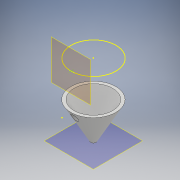
# Autodesk Inventor part: EMBOUT
Saved by Autodesk Inventor 2018 (Build 220112000, 112)
## iProperties
Created: 2018-05-14
Part Number: EMBOUT
Material: Générique
Document SubType Name: Modeling
Designer: Dimitri
Density: 1 g/cm^3
Appearance: Par défaut
Author: Dimitri
Autodesk Inventor part; units mm, degrees
ref_plane "YZ Plane" through (0, 0, 0) normal (1, 0, 0) x (0, 1, 0)
ref_plane "XZ Plane" through (0, 0, 0) normal (0, 1, 0) x (-1, 0, 0)
ref_plane "XY Plane" through (0, 0, 0) normal (0, 0, 1) x (1, 0, 0)
sketch "Esquisse1" plane through (0, 0, 0) normal (0, 0, 1) x (1, 0, 0)
  circle A0 centre (0, 0) radius 12.5
  dimension "d0" = 25
  constraints: 1 centre point, 1 coincident
  measures "d0" diameter of A0
extrude "Extrusion1" add sketch "Esquisse1" along normal blind 20
shell "Coque1" thickness 1.5 removed faces 1 at (2.488, -2.432, 20)
ref_plane "Plan de construction1" through (0, 0, -20) normal (0, 0, -1) x (-1, 0, 0)
sketch "Esquisse2" plane through (0, 0, -20) normal (0, 0, -1) x (-1, 0, 0)
  circle A0 centre (0, 0) radius 1.5
  dimension "d5" = 3
  constraints: 1 centre point, 1 coincident
  measures "d5" diameter of A0
loft "Lissage1" add profiles "Esquisse2" section 2 edges at (-12.5, 0, 0)
shell "Coque2" thickness 1.5 removed faces 1 at (0.3952, -0.1996, -20)
sketch "Esquisse3" plane through (0, 0, -20) normal (0, 0, -1) x (-1, 0, 0)
  circle A0 centre (0, 0) radius 1.1
  dimension "d11" = 2.2
  constraints: 1 centre point, 1 coincident
  measures "d11" diameter of A0
extrude "Extrusion2" cut sketch "Esquisse3" against normal blind 10
sketch "Esquisse4" plane through (0, 0, 20) normal (0, 0, 1) x (1, 0, 0)
  circle A0 centre (0, 0) radius 12.5 projected
  point P0 (0, -12.5)
  constraints: 1 vertical alignment, 1 other
ref_plane "Plan de construction2" through (0, -12.5, 20) normal (0, -1, 0) x (1, 0, 0)
sketch "Esquisse5" plane through (0, -12.5, 20) normal (0, -1, 0) x (1, 0, 0)
  circle A0 centre (0, -23.4729) radius 1
  circle A1 centre (0, -23.4729) radius 1.5
  point P0 (0, -20)
  dimension "d14" = 2
  dimension "d15" = 3
  constraints: 2 centre point, 1 coincident
  measures "d14" diameter of A0
  measures "d15" diameter of A1
extrude "Extrusion3" add sketch "Esquisse5" along normal mid plane 10
sketch "Esquisse6" plane through (0, -17.5, -3.4729) normal (0, -1, 0) x (1, 0, 0)
  circle A0 centre (0, 0) radius 1
  point P0 (0, 3.4729)
  constraints: 1 centre point
extrude "Extrusion4" cut sketch "Esquisse6" against normal blind 15
sketch "Esquisse7" plane through (0, -17.5, -3.4729) normal (0, -1, 0) x (1, 0, 0)
  point P0 (0, 3.4729)
sketch "Esquisse8" plane through (0, -17.5, -3.4729) normal (0, -1, 0) x (1, 0, 0)
  circle A0 centre (0, 0) radius 1 projected
  circle A1 centre (0, 0) radius 2
  point P0 (0, 3.4729)
  dimension "d20" = 4
  constraints: 1 centre point, 1 coincident
  measures "d20" diameter of A1
extrude "Extrusion5" cut sketch "Esquisse8" against normal blind 10
sketch "Esquisse9" plane through (0, 0, 0) normal (0, 0, -1) x (-1, 0, 0)
  circle A0 centre (0, 0) radius 20.0804
  constraints: 1 centre point, 1 coincident
extrude "Extrusion6" cut sketch "Esquisse9" against normal blind 20
